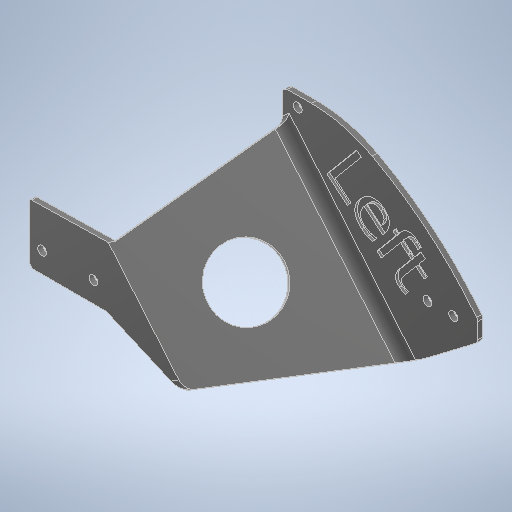
# Autodesk Inventor part: 3D_side-accessory
Saved by Autodesk Inventor 2025.1 (Build 291241020, 241B)
## iProperties
Created: 2024-09-24
Part Number: 3D_side-accessory
Material: 一般
Document SubType Name: Modeling
Designer: 8326d
Density: 1 g/cm^3
Appearance: 滑らか - 黒
Author: 8326d
Autodesk Inventor part; units mm, degrees
ref_plane "YZ Plane" through (0, 0, 0) normal (1, 0, 0) x (0, 1, 0)
ref_plane "XZ Plane" through (0, 0, 0) normal (0, 1, 0) x (-1, 0, 0)
ref_plane "XY Plane" through (0, 0, 0) normal (0, 0, 1) x (1, 0, 0)
ref_plane "作業平面1" through (0, 0, 0) normal (0, 0, 1) x (1, 0, 0)
sketch "スケッチ1" plane through (0, 0, 0) normal (0, 0, 1) x (1, 0, 0)
  arc A0 (102.0393, 80.548) -> (61.4446, 114.5625) centre (0, 0) ccw projected
  arc A1 (102.4695, 79.3088) -> (102.0393, 80.548) centre (100.4695, 79.3088) ccw projected
  line L0 (102.4695, 73.1789) -> (102.4695, 79.3088) projected
  arc A2 (101.6775, 71.5849) -> (102.4695, 73.1789) centre (100.4695, 73.1789) ccw projected
  line L1 (60.792, 40.6002) -> (101.6775, 71.5849) projected
  circle A3 centre (92.9695, 76.5) radius 1.75 projected
  circle A4 centre (82.9695, 76.5) radius 1.75 projected
  arc A5 (61.4446, 114.5625) -> (37.812, 120.5) centre (37.812, 70.5) ccw projected
  circle A6 centre (32.5, 116.5) radius 1.75 projected
  line L2 (37.812, 120.5) -> (-37.812, 120.5) projected
  line L3 (74.6235, 51.0823) -> (26.5, 108.4337)
  line L4 (26.5, 108.4337) -> (26.5, 120.5)
  point P0 (0, 0)
  dimension "d0" = 50
  dimension "d1" = 90
  dimension "d2" = 6
  constraints: 4 end point, 2 point on line, 1 perpendicular
  measures "d0" angle of L2 L3
  measures "d1" distance from line of point (0, 0) L3
  measures "d2" distance from line of A6.centre L4
extrude "押し出し1" add sketch "スケッチ1" along normal blind 2
ref_plane "作業平面2" through (26.5, 108.4337, 0) normal (-0.7198463, -0.6040228, -0.3420201) x (0.6427876, -0.7660444, 0)
sketch "スケッチ2" plane through (26.5, 108.4337, 0) normal (-0.7198463, -0.6040228, -0.3420201) x (0.6427876, -0.7660444, 0)
  line L0 (7.112, 60.7019) -> (54.1566, 74.2031) projected
  line L1 (0, 0) -> (74.8669, 0) projected
  line L2 (0, 0) -> (7.112, 60.7019)
  line L3 (74.8669, 0) -> (48.4548, 72.5668)
  point P0 (66.0311, 30.7818)
  dimension "d6" = 70
  constraints: 4 end point, 1 point on line
  measures "d6" angle of L1 L3
extrude "押し出し2" add sketch "スケッチ2" against normal blind 2
sketch "スケッチ3" plane through (0, 0, 0) normal (1, 0, 0) x (0, 1, 0)
  line L0 (90.8485, 57.7251) -> (56.5697, 68.8745) projected
  line L1 (109.2082, 2) -> (90.8485, 57.7251) projected
  line L2 (55.3616, 68.1905) -> (56.5697, 68.8745) projected
  line L3 (51.0823, 0) -> (55.3616, 68.1905) projected
  line L4 (28.0876, 56.9615) -> (89.5, 56.9615) projected
  line L5 (89.5, 56.9615) -> (91.1001, 56.9615)
  point P0 (0, 0)
  point P1 (54.657, 56.9615)
  constraints: 2 end point, 1 horizontal, 1 point on line
extrude "押し出し3" cut sketch "スケッチ3" along normal through all
sketch "スケッチ4" plane through (46.3606, 55.8221, 56.9615) normal (0, 0, 1) x (0.7660444, 0.6427876, 0)
  line L0 (-2.1284, 0.2649) -> (-2.1284, 45.9669)
  line L1 (-23.9484, 65.3639) -> (-2.4992, 47.3658)
  arc A0 (-2.3759, 45.957) -> (-2.4992, 47.3658) centre (-3.1419, 46.5998) ccw
  line L2 (-2.3759, 45.957) -> (-41.8511, -1.0876)
  circle A1 centre (-15.2051, 38.4463) radius 1.75
  circle A2 centre (-30.526, 51.3021) radius 1.75
  line L3 (-64.8324, 18.196) -> (-25.3572, 65.2406)
  arc A3 (-23.9484, 65.3639) -> (-25.3572, 65.2406) centre (-24.5912, 64.5979) ccw
  line L4 (-2.1284, 45.9669) -> (0, 46.0522)
  line L5 (0, 46.0522) -> (0, 0)
  line L6 (0, 0) -> (-2.1284, 0.2649)
  line L7 (-39.4986, 48.3877) -> (-16.5172, 29.104)
  line L8 (-2.1284, 0.2649) -> (-16.5172, 29.104)
  line L9 (0, 46.0522) -> (-23.9635, 65.3763)
  point P0 (-71.3961, -12.9621)
extrude "押し出し4" add sketch "スケッチ4" along normal blind 2
ref_plane "作業平面3" through (66.8878, 46.8855, 2) normal (-0.1745919, 0.2698363, 0.9469456) x (-0.8395817, -0.5432335, 0)
sketch "スケッチ5" plane through (66.8878, 46.8855, 2) normal (-0.1745919, 0.2698363, 0.9469456) x (-0.8395817, -0.5432335, 0)
  line L0 (-8.6901, 0) -> (-8.7746, 0.6428) projected
  line L1 (-8.7746, 0.6428) -> (-42.6264, -1.7407) projected
  line L2 (12.3796, 0) -> (-10.1013, 0) projected
  line L3 (-10.1013, 0) -> (-17.904, 0)
  point P0 (81.6275, 2.2251)
  constraints: 2 end point, 1 horizontal, 1 point on line
extrude "押し出し5" cut sketch "スケッチ5" against normal through all
sketch "スケッチ6" plane through (26.6415, 108.265, 2) normal (-0.6689091, 0.7352575, 0.1093487) x (0.7400084, 0.6725835, 0.0043555)
  line L0 (-18.6187, -55.3752) -> (-18.61, -57.3632) projected
  line L1 (-20.4318, -62.4029) -> (-18.61, -57.3632) projected
  line L2 (-18.61, -57.3632) -> (-41.79, -55.2485) projected
  line L3 (-18.6187, -55.3752) -> (-21.1556, -62.393)
  line L4 (-22.548, -62.3739) -> (-20.4318, -62.4029) projected
  line L5 (1.4015, 0.0061) -> (-18.6187, -55.3752) projected
  point P0 (-92.5409, -5.2141)
  constraints: 2 end point, 1 collinear, 1 point on line
extrude "押し出し6" cut sketch "スケッチ6" along normal through all both and the other way through all
fillet "フィレット1" radius 5 1 edges at (51.5235, 80.7905, 2)
fillet "フィレット2" radius 2 2 edges at (28.9741, 110.3871, 2) (27.1599, 108.7366, 2)
fillet "フィレット3" radius 2 3 edges at (26.5, 120.5, 1) (-15, 67.5, 57.9615) (15, 67.5, 57.9615)
fillet "フィレット4" radius 5 1 edges at (45.1523, 55.0403, 58.9615)
sketch "スケッチ7" plane through (27.9397, 109.6417, 0.684) normal (0.7198463, 0.6040228, 0.3420201) x (0.2620026, 0.2198463, -0.9396926)
  line L0 (-0.203, -74.793) -> (-0.203, 1.7697) projected
  point P0 (-30.7818, -66.0311)
  point P1 (-32.203, -34.0311)
  dimension "d23" = 32
  dimension "d24" = 32
  measures "d23" distance from line of L0 point (-32.203, -34.031)
  measures "d24" vertical distance of point (-30.782, -66.031) point (-32.203, -34.031)
hole "穴1" at (41.3772, 76.4926, 30.945) direction (-0.7198463, -0.6040228, -0.3420201) diameter 25 end through all
sketch "スケッチ8" plane through (0, 0, 2) normal (0, 0, 1) x (1, 0, 0)
  line L0 (54.5674, 115.4475) -> (77.4059, 96.2838) construction
  line L1 (77.4059, 96.2838) -> (7.0998, 12.4963) construction
  line L2 (7.0998, 12.4963) -> (-15.7386, 31.6601) construction
  line L3 (-15.7386, 31.6601) -> (54.5674, 115.4475) construction
  line L4 (51.7928, 93.0788) -> (43.8033, 99.7827)
  line L5 (43.8033, 99.7827) -> (55.3735, 113.5715)
  line L6 (55.3735, 113.5715) -> (57.206, 112.0338)
  line L7 (57.206, 112.0338) -> (47.0048, 99.8764)
  line L8 (47.0048, 99.8764) -> (53.1617, 94.7102)
  line L9 (53.1617, 94.7102) -> (51.7928, 93.0788)
  spline S0 degree 2 poles (57.3952, 87.9779) (54.9146, 90.0594) (54.5228, 95.1295) (56.6793, 97.6996) knots 0 0 0 1 2 2 2
  spline S1 degree 2 poles (56.6793, 97.6996) (58.7983, 100.2249) (63.9594, 100.9974) (66.0936, 99.2065) knots 0 0 0 1 2 2 2
  spline S2 degree 2 poles (66.0936, 99.2065) (67.0546, 98.4002) (68.0719, 96.5945) (68.1225, 95.5428) knots 0 0 0 1 2 2 2
  spline S3 degree 2 poles (68.1225, 95.5428) (68.1843, 94.4818) (67.3419, 92.2752) (66.3012, 91.0349) knots 0 0 0 1 2 2 2
  line L10 (66.3012, 91.0349) -> (65.5042, 90.0851)
  line L11 (65.5042, 90.0851) -> (58.3416, 96.0952)
  spline S4 degree 2 poles (58.3416, 96.0952) (56.8321, 94.2962) (57.039, 90.8665) (58.648, 89.5163) knots 0 0 0 1 2 2 2
  spline S5 degree 2 poles (58.648, 89.5163) (59.2179, 89.0381) (60.5398, 88.3669) (61.1555, 88.193) knots 0 0 0 1 2 2 2
  spline S6 degree 2 poles (61.1555, 88.193) (61.8124, 88.0227) (62.7886, 87.8699) (63.1509, 87.8706) knots 0 0 0 1 2 2 2
  line L12 (63.1509, 87.8706) -> (63.2515, 87.7862)
  line L13 (63.2515, 87.7862) -> (61.6576, 85.8866)
  spline S7 degree 2 poles (61.6576, 85.8866) (61.2527, 86.0168) (60.0364, 86.4281) (59.5945, 86.6276) knots 0 0 0 1 2 2 2
  spline S8 degree 2 poles (59.5945, 86.6276) (58.9697, 86.9042) (58.021, 87.4528) (57.3952, 87.9779) knots 0 0 0 1 2 2 2
  spline S9 degree 2 poles (64.9215, 92.84) (65.4899, 93.5627) (66.062, 94.8345) (66.0733, 95.4153) knots 0 0 0 1 2 2 2
  spline S10 degree 2 poles (66.0733, 95.4153) (66.0997, 96.0595) (65.4969, 97.27) (64.7929, 97.8607) knots 0 0 0 1 2 2 2
  spline S11 degree 2 poles (64.7929, 97.8607) (64.1001, 98.442) (62.781, 98.8443) (62.0412, 98.7795) knots 0 0 0 1 2 2 2
  spline S12 degree 2 poles (62.0412, 98.7795) (61.3032, 98.6943) (60.0665, 98.0373) (59.4574, 97.4249) knots 0 0 0 1 2 2 2
  line L14 (59.4574, 97.4249) -> (64.9215, 92.84)
  line L15 (79.1998, 91.7699) -> (79.1104, 91.8449)
  spline S13 degree 2 poles (79.1104, 91.8449) (78.9508, 92.1312) (78.2104, 93.019) (77.864, 93.3097) knots 0 0 0 1 2 2 2
  spline S14 degree 2 poles (77.864, 93.3097) (76.769, 94.2285) (75.0053, 94.0328) (73.9176, 92.7366) knots 0 0 0 1 2 2 2
  line L16 (73.9176, 92.7366) -> (73.627, 92.3902)
  line L17 (73.627, 92.3902) -> (76.5099, 89.9712)
  line L18 (76.5099, 89.9712) -> (75.3004, 88.5297)
  line L19 (75.3004, 88.5297) -> (72.4733, 90.9019)
  line L20 (72.4733, 90.9019) -> (65.0005, 81.9962)
  line L21 (65.0005, 81.9962) -> (63.2574, 83.4588)
  line L22 (63.2574, 83.4588) -> (70.7302, 92.3646)
  line L23 (70.7302, 92.3646) -> (69.5569, 93.3491)
  line L24 (69.5569, 93.3491) -> (70.7664, 94.7905)
  line L25 (70.7664, 94.7905) -> (71.9397, 93.806)
  line L26 (71.9397, 93.806) -> (72.2303, 94.1524)
  spline S15 degree 2 poles (72.2303, 94.1524) (73.7868, 96.0073) (77.2173, 96.442) (78.8934, 95.0356) knots 0 0 0 1 2 2 2
  spline S16 degree 2 poles (78.8934, 95.0356) (79.3739, 94.6324) (80.2169, 93.7536) (80.5406, 93.3678) knots 0 0 0 1 2 2 2
  line L27 (80.5406, 93.3678) -> (79.1998, 91.7699)
  spline S17 degree 2 poles (72.0725, 75.7193) (70.6534, 76.91) (70.4151, 79.8711) (71.8871, 81.6254) knots 0 0 0 1 2 2 2
  line L28 (71.8871, 81.6254) -> (76.6971, 87.3577)
  line L29 (76.6971, 87.3577) -> (75.5238, 88.3422)
  line L30 (75.5238, 88.3422) -> (76.7334, 89.7836)
  line L31 (76.7334, 89.7836) -> (77.9066, 88.7992)
  line L32 (77.9066, 88.7992) -> (80.4007, 91.7715)
  line L33 (80.4007, 91.7715) -> (82.1439, 90.3088)
  line L34 (82.1439, 90.3088) -> (79.6498, 87.3365)
  line L35 (79.6498, 87.3365) -> (82.8568, 84.6455)
  line L36 (82.8568, 84.6455) -> (81.6472, 83.2041)
  line L37 (81.6472, 83.2041) -> (78.4403, 85.895)
  line L38 (78.4403, 85.895) -> (74.3054, 80.9673)
  spline S18 degree 2 poles (74.3054, 80.9673) (73.6491, 80.1851) (72.983, 79.2778) (72.8635, 78.7496) knots 0 0 0 1 2 2 2
  spline S19 degree 2 poles (72.8635, 78.7496) (72.748, 78.2943) (73.1801, 77.3796) (73.7835, 76.8733) knots 0 0 0 1 2 2 2
  spline S20 degree 2 poles (73.7835, 76.8733) (74.2081, 76.517) (75.2171, 76.1083) (75.4615, 76.0365) knots 0 0 0 1 2 2 2
  line L39 (75.4615, 76.0365) -> (75.5621, 75.9521)
  line L40 (75.5621, 75.9521) -> (74.2494, 74.3877)
  spline S21 degree 2 poles (74.2494, 74.3877) (73.6453, 74.6662) (72.5083, 75.3536) (72.0725, 75.7193) knots 0 0 0 1 2 2 2
  point P0 (0, 0)
  constraints: 2 other
extrude "押し出し7" cut sketch "スケッチ8" against normal blind 1
